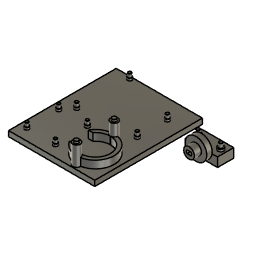
Scidrom lidar frame v1 (Autodesk Fusion 360 design; units mm, degrees)
Autodesk Fusion 360 part; units mm, degrees
note: some values were not read from the file. Set by a fixed rule: which sketch regions a step uses.
sketch "Sketch1" plane through (0, 0, 0) normal (0, 0, 1) x (1, 0, 0)
  line L0 (-46.7846, 50.2138) -> (33.2154, 50.2138)
  line L1 (33.2154, 50.2138) -> (33.2154, -39.7862)
  line L2 (33.2154, -39.7862) -> (-46.7846, -39.7862)
  line L3 (-46.7846, -39.7862) -> (-46.7846, 50.2138)
  dimension "d1" = 80
  dimension "d2" = 90
  constraint horizontal L0
  constraint vertical L1
  constraint horizontal L2
  constraint vertical L3
  measures "d1" distance of L0.start L0.end
  measures "d2" distance of L0.start L2.end
extrude "Extrude1" add sketch "Sketch1" along normal blind 5 makes body 1
sketch "Sketch2" plane through (0, 0, 5) normal (0, 0, 1) x (-1, 0, 0)
  line L0 (-33.2154, 39.7862) -> (-33.2154, -50.2138)
  line L1 (-33.2154, -50.2138) -> (46.7846, -50.2138)
  line L2 (46.7846, -50.2138) -> (46.7846, 39.7862)
  circle A0 centre (32.7846, 0.5862) radius 1.575
  circle A1 centre (32.7846, 0.5862) radius 2
  circle A2 centre (-18.7154, -32.2138) radius 1.575
  circle A3 centre (-18.7154, -4.2138) radius 1.575
  circle A4 centre (31.7846, -47.7138) radius 1.575
  circle A5 centre (31.7846, -47.7138) radius 2
  circle A6 centre (-18.7154, -32.2138) radius 2
  circle A7 centre (-18.7154, -4.2138) radius 2
  dimension "d5" = 3.15
  dimension "d6" = 50.8
  dimension "d7" = 14
  dimension "d8" = 4
  dimension "d9" = 3.15
  dimension "d10" = 65.5
  dimension "d11" = 18
  dimension "d12" = 3.15
  dimension "d13" = 46
  dimension "d14" = 65.5
  dimension "d15" = 3.15
  dimension "d16" = 15
  dimension "d17" = 2.5
  dimension "d18" = 4
  dimension "d19" = 4
  dimension "d20" = 4
  constraint concentric A0 A1
  constraint concentric A4 A5
  constraint concentric A2 A6
  constraint concentric A3 A7
  measures "d5" diameter of A0
  measures "d6" distance of L1 A0.centre
  measures "d7" distance of L2 A0.centre
  measures "d8" diameter of A1
  measures "d9" diameter of A2
  measures "d10" distance of L2 A2.centre
  measures "d11" distance of L1 A2.centre
  measures "d12" diameter of A3
  measures "d13" distance of L1 A3.centre
  measures "d14" distance of L2 A3.centre
  measures "d15" diameter of A4
  measures "d16" distance of L2 A4.centre
  measures "d17" distance of L1 A4.centre
  measures "d18" diameter of A5
  measures "d19" diameter of A6
  measures "d20" diameter of A7
extrude "Extrude2" add sketch "Sketch2" along normal blind 2.1 contours A1 bodies 1
extrude "Extrude3" add 1 faces at (-33.1178, -1.0749, 5) along direction (0, 0, 1) blind 5.6 on bodies 1 bodies 1
fillet "Fillet1" radius 0.3 1 edges at (-31.3161, -0.0167, 10.6) on bodies 1
extrude "Extrude4" add sketch "Sketch2" along normal blind 2.1 contours A5 | A6 | A7 bodies 1
extrude "Extrude5" add sketch "Sketch2" along normal blind 5.6 contours A2 | A3 | A4 bodies 1
fillet "Fillet2" radius 0.3 3 edges at (-30.3161, 48.2833, 10.6) (20.1839, 32.7833, 10.6) (20.1839, 4.7833, 10.6) on bodies 1
sketch "Sketch3" plane through (0, 0, 5) normal (0, 0, 1) x (-1, 0, 0)
  line L0 (46.7846, -50.2138) -> (46.7846, 39.7862)
  line L1 (-33.2154, 39.7862) -> (-33.2154, -50.2138)
  line L2 (46.7846, 4.7862) -> (-33.2154, 4.7862)
  line L3 (-33.2154, -50.2138) -> (46.7846, -50.2138)
  dimension "d33" = 55
  constraint coincident L0 L2.start
  constraint coincident L1 L2.end
  constraint perpendicular L1 L2
  measures "d33" distance of L2 L3
sketch "Sketch4" plane through (0, 0, 5) normal (0, 0, 1) x (-1, 0, 0)
  circle A0 centre (40, 10) radius 2
  circle A1 centre (13.4, 10) radius 2
  circle A2 centre (40, 39.6) radius 2
  circle A3 centre (13.4, 39.6) radius 2
  dimension "d34" = 4
  dimension "d37" = -26.6
  dimension "d38" = 29.6
  measures "d34" diameter of A0
extrude "Extrude6" add 1 faces at (6.5488, -39.7862, 1.6667) along direction (0, -1, 0) blind 3 on bodies 1 bodies 1
sketch "Sketch5" plane through (0, 0, 5) normal (0, 0, 1) x (-1, 0, 0)
  circle A0 centre (-18.7154, -32.2138) radius 2
  circle A1 centre (32.7846, 0.5862) radius 2
  line L0 (-33.2154, -50.2138) -> (46.7846, -50.2138)
  line L1 (46.7846, -50.2138) -> (46.7846, 42.7862)
  circle A2 centre (-18.7154, -4.2138) radius 2
  circle A3 centre (31.7846, -47.7138) radius 2
extrude "Extrude7" add sketch "Sketch4" along normal blind 2 bodies 1
sketch "Sketch6" plane through (0, 0, 7) normal (0, 0, 1) x (-1, 0, 0)
  circle A0 centre (40, 10) radius 2
  circle A1 centre (40, 10) radius 1.475
  circle A2 centre (13.4, 10) radius 1.475
  circle A3 centre (13.4, 39.6) radius 1.475
  circle A4 centre (40, 39.6) radius 2
  circle A5 centre (40, 39.6) radius 1.475
  dimension "d43" = 2.95
  dimension "d44" = 2.95
  dimension "d45" = 2.95
  dimension "d46" = 2.95
  constraint concentric A0 A1
  constraint concentric A4 A5
  measures "d43" diameter of A1
  measures "d44" diameter of A2
  measures "d45" diameter of A3
  measures "d46" diameter of A5
extrude "Extrude8" add sketch "Sketch6" along normal blind 3.5 contours A1 | A2 | A3 | A5 bodies 1
fillet "Fillet3" radius 0.3 4 edges at (-38.6248, -9.4666, 10.5) (-12.0248, -9.4666, 10.5) (-12.0248, -39.0666, 10.5) (-38.6248, -39.0666, 10.5) on bodies 1
sketch "Sketch7" plane through (0, 0, 5) normal (0, 0, 1) x (-1, 0, 0)
  circle A0 centre (-12, 23) radius 17.5
  circle A1 centre (-12, 23) radius 14.005
  dimension "d51" = 35
  dimension "d52" = 28.01
  constraint concentric A0 A1
  measures "d51" diameter of A0
  measures "d52" diameter of A1
sketch "Sketch8" plane through (0, 0, 5) normal (0, 0, 1) x (-1, 0, 0)
  circle A0 centre (-12, 23) radius 14.005
  line L0 (-11.9996, 37.005) -> (-11.9996, 8.995)
  line L1 (-11.9996, 30.405) -> (-11.9996, 37.005)
  line L2 (-11.9996, 15.595) -> (-11.9996, 8.995)
  line L3 (5.9968, 31.905) -> (-1.9489, 31.905)
  line L4 (-1.9489, 31.905) -> (-1.9489, 14.305)
  line L5 (-1.9489, 14.305) -> (5.9968, 14.305)
  line L6 (5.9968, 14.305) -> (5.9968, 31.905)
  dimension "d53" = 6.6
  dimension "d54" = 6.6
  dimension "d55" = 17.6
  constraint coincident A0 L0.start
  constraint coincident A0 L0.end
  constraint vertical L1
  constraint vertical L2
  constraint horizontal L3
  constraint vertical L4
  constraint horizontal L5
  constraint vertical L6
  measures "d53" distance of L0.start L1.start
  measures "d54" distance of L0.end L2.start
  measures "d55" distance of L3 L5
extrude "Extrude9" add sketch "Sketch7" along normal blind 7 bodies 1
extrude "Extrude10" cut sketch "Sketch8" along normal blind 7 contours A0 L3 L5 L6 bodies 1
sketch "Sketch9" plane through (0, 0, 5) normal (0, 0, 1) x (-1, 0, 0)
  circle A0 centre (-12, 45.5) radius 3.5
  dimension "d60" = 7
  measures "d60" diameter of A0
extrude "Extrude11" add 1 faces at (6.5488, -42.7862, 1.6667) along direction (0, -1, 0) blind 7 on bodies 1 bodies 1
move_face "MoveFace1" to x (1, 0, 0) y (0, 1, 0) z (0, 0, 1) at (0, -5, 0) 5 faces at (1.6468, -32.4314, 7.3333) (-0.3816, -14.305, 7.3333) (-0.0522, -33.9662, 12) (-2.2471, -12.8379, 7.3333) (-1.6464, -31.905, 7.3333) on bodies 1
sketch "Sketch10" plane through (0, 0, 5) normal (0, 0, 1) x (-1, 0, 0)
  circle A0 centre (31.7846, -47.7138) radius 2
  circle A1 centre (-18.7154, -4.2138) radius 2
  line L0 (-33.2154, 49.7862) -> (-33.2154, -50.2138)
  line L1 (-33.2154, -50.2138) -> (46.7846, -50.2138)
  line L2 (46.7846, -50.2138) -> (46.7846, 49.7862)
  line L3 (46.7846, 49.7862) -> (-33.2154, 49.7862)
  circle A2 centre (32.7846, 0.5862) radius 2
  circle A3 centre (-18.7154, -32.2138) radius 2
  circle A4 centre (13.4, 10) radius 2
  circle A5 centre (13.4, 39.6) radius 2
  circle A6 centre (40, 10) radius 2
  circle A7 centre (40, 39.6) radius 2
  arc A8 (-1.1907, 36.905) -> (-1.0211, 19.305) centre (-12, 28) ccw
  line L4 (-1.0211, 19.305) -> (3.1871, 19.305)
  arc A9 (3.0649, 36.905) -> (3.1871, 19.305) centre (-12, 28) ccw
  line L5 (3.0649, 36.905) -> (-1.1907, 36.905)
extrude "Extrude12" add sketch "Sketch9" along normal blind 18 bodies 1
sketch "Sketch11" plane through (0, 0, 5) normal (0, 0, 1) x (-1, 0, 0)
  circle A0 centre (-12, 10.5) radius 3.5
  arc A1 (3.0649, 36.905) -> (3.1871, 19.305) centre (-12, 28) ccw
  dimension "d66" = 7
  constraint coincident A0.centre A1
  measures "d66" diameter of A0
extrude "Extrude13" add sketch "Sketch11" along normal blind 18 bodies 1
sketch "Sketch12" plane through (0, 0, 23) normal (0, 0, 1) x (-1, 0, 0)
  circle A0 centre (-12, 45.5) radius 3.5
  circle A1 centre (-12, 45.5) radius 1.975
  circle A2 centre (-12, 10.5) radius 2
  dimension "d69" = 3.95
  dimension "d70" = 4
  constraint concentric A0 A1
  measures "d69" diameter of A1
  measures "d70" diameter of A2
extrude "Extrude14" add sketch "Sketch12" along normal blind 2 contours A1 | A2 bodies 1
fillet "Fillet4" radius 0.1 2 edges at (13.8647, -9.7768, 25) (13.8413, -44.7858, 25) on bodies 1
sketch "Sketch13" plane through (0, 0, 0) normal (0, 0, 1) x (1, 0, 0)
sketch "Sketch14" plane through (0, 0, 0) normal (0, 0, 1) x (1, 0, 0)
  circle A0 centre (60, 41) radius 2.5
  circle A1 centre (60, 41) radius 5
  line L0 (60, 39.5) -> (62, 39.5)
  line L1 (60, 39.5) -> (58, 39.5)
  line L2 (60, 42.5) -> (58, 42.5)
  line L3 (60, 42.5) -> (62, 42.5)
  dimension "d75" = 5
  constraint concentric A0 A1
  constraint coincident A0 L0.end
  constraint horizontal L0
  constraint coincident A0 L1.end
  constraint parallel L0 L1
  constraint coincident A0 L2.end
  constraint parallel L0 L2
  constraint coincident A0 L3.end
  constraint parallel L2 L3
  measures "d75" diameter of A0
extrude "Extrude15" add sketch "Sketch14" along normal blind 6.5 separate body contours A0 L2 L3 | A0 L0 L1 | A1 makes body 2
sketch "Sketch15" plane through (0, 0, 6.5) normal (0, 0, 1) x (-1, 0, 0)
  arc A0 (-58, -42.5) -> (-58, -39.5) centre (-60, -41) ccw
  line L0 (-58, -42.5) -> (-62, -42.5)
  arc A1 (-62, -39.5) -> (-62, -42.5) centre (-60, -41) ccw
  line L1 (-62, -39.5) -> (-58, -39.5)
  circle A2 centre (-60, -41) radius 5
  circle A3 centre (-60, -41) radius 10
  dimension "d79" = 20
  constraint concentric A0 A3
  measures "d79" diameter of A3
extrude "Extrude16" add sketch "Sketch15" along normal blind 5 contours A0 L0 A1 L1 | A2 | A3 bodies 2
sketch "Sketch16" plane through (0, 0, 11.5) normal (0, 0, 1) x (-1, 0, 0)
  circle A0 centre (-60, -41) radius 10
  line L0 (-50, -41) -> (-70, -41)
  line L1 (-45, -47.5) -> (-75, -47.5)
  line L2 (-75, -47.5) -> (-75, -42.5)
  line L3 (-75, -42.5) -> (-45, -42.5)
  line L4 (-45, -42.5) -> (-45, -47.5)
  line L5 (-45, -47.5) -> (-75, -42.5) construction
  line L6 (-75, -47.5) -> (-45, -42.5) construction
  point P0 (-60, -45)
  dimension "d82" = 30
  dimension "d83" = 5
  constraint coincident A0 L0.start
  constraint coincident A0 L0.end
  constraint horizontal L0
  constraint horizontal L1
  constraint perpendicular L1 L2
  constraint parallel L1 L3
  constraint parallel L2 L4
  constraint coincident L5 P0
  constraint coincident L6 P0
  measures "d82" distance of L2.end L3.end
  measures "d83" distance of L1.end L2.end
extrude "Extrude17" add sketch "Sketch16" along normal blind 15 contours A0 L1 L3 L4 | A0 L1 L3 | A0 L1 L2 L3 bodies 2
sketch "Sketch17" plane through (0, 42.5, 0) normal (0, -1, 0) x (1, 0, 0)
  line L0 (69.8869, 11.5) -> (75, 11.5)
  line L1 (75, 11.5) -> (75, 26.5)
  line L2 (75, 26.5) -> (45, 26.5)
  line L3 (45, 26.5) -> (45, 11.5)
  line L4 (45, 11.5) -> (50.1131, 11.5)
  line L5 (50.1131, 11.5) -> (69.8869, 11.5)
  line L6 (68, 25) -> (52, 25)
  line L7 (52, 25) -> (52, 13)
  line L8 (52, 13) -> (68, 13)
  line L9 (68, 13) -> (68, 25)
  line L10 (68, 25) -> (52, 13) construction
  line L11 (52, 25) -> (68, 13) construction
  line L12 (52, 19) -> (49.5, 19)
  circle A0 centre (49.5, 19) radius 2.75
  circle A1 centre (70.5, 19) radius 2.75
  circle A2 centre (49.5, 19) radius 1.625
  circle A3 centre (70.5, 19) radius 1.625
  point P0 (60, 19)
  dimension "d86" = 16
  dimension "d87" = 12
  dimension "d88" = 2.5
  dimension "d89" = 5.5
  dimension "d92" = 21
  dimension "d93" = 0
  dimension "d94" = 3.25
  dimension "d95" = 3.25
  constraint horizontal L6
  constraint perpendicular L6 L7
  constraint parallel L6 L8
  constraint parallel L7 L9
  constraint coincident L10 P0
  constraint coincident L11 P0
  constraint midpoint L7 L12.start
  constraint perpendicular L7 L12
  constraint coincident L12.end A0.centre
  constraint concentric A0 A2
  constraint concentric A1 A3
  measures "d86" distance of L7.end L8.end
  measures "d87" distance of L6.end L7.end
  measures "d88" distance of L12.start L12.end
  measures "d89" diameter of A0
  measures "d94" diameter of A2
  measures "d95" diameter of A3
extrude "Extrude18" add sketch "Sketch17" along normal blind 2 contours L9 A1 | L9 A1 | L7 A0 | L7 A0 bodies 2
extrude "Extrude19" add 2 faces at (49.3722, 42.5, 19.3588) (69.9239, 42.5, 18.5406) along direction (0, -1, 0) blind 6 on bodies 2 bodies 2
extrude "Extrude20" add 1 faces at (62.5331, 47.5, 21.5) along direction (0, 1, 0) blind 3.5 on bodies 2 bodies 2
move_body "Move1" bodies 2 to x (1, 0, 0) y (0, 0, -1) z (0, 1, 0) at (0, 31, 51)
move_body "Move2" bodies 2 to x (1, 0, 0) y (0, 1, 0) z (0, 0, 1) at (0, 110, 0)
move_body "Move3" bodies 2 to x (1, 0, 0) y (0, 1, 0) z (0, 0, 1) at (0, -130, 0)
fillet "Fillet5" radius 0.2 2 edges at (47.985, 29.4124, 14.5) (68.985, 29.4124, 14.5) on bodies 2
equation "d23 = 2.1 mm + 3.5 mm"
equation "d29 = 2.1 mm + 3.5 mm"
equation "d55 = 14.6 mm + 3 mm"
equation "d88 = 5 mm / 2"
equation "d98 = 2 mm + 4 mm"
